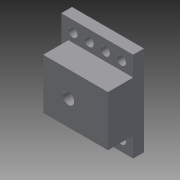
# Autodesk Inventor part: end limit holder
Saved by Autodesk Inventor 2013 SP2 (Build 170200200, 200)
## iProperties
Created: 2017-05-27
Part Number: end limit holder
Material: Generic
Document SubType Name: Modeling
Designer: hdv
Density: 1 g/cm^3
Author: hdv
Autodesk Inventor part; units mm, degrees
ref_plane "YZ Plane" through (0, 0, 0) normal (1, 0, 0) x (0, 1, 0)
ref_plane "XZ Plane" through (0, 0, 0) normal (0, 1, 0) x (-1, 0, 0)
ref_plane "XY Plane" through (0, 0, 0) normal (0, 0, 1) x (1, 0, 0)
sketch "Sketch1" plane through (0, 0, 0) normal (0, 0, 1) x (1, 0, 0)
  line L0 (0, 0) -> (20, 0)
  line L1 (20, 0) -> (20, 25)
  line L2 (20, 25) -> (0, 25)
  line L3 (0, 25) -> (0, 0)
  line L4 (5, 16.5) -> (17, 16.5)
  line L5 (17, 16.5) -> (17, 8.5)
  line L6 (17, 8.5) -> (5, 8.5)
  line L7 (5, 8.5) -> (5, 16.5)
  point P0 (17, 12.5)
  point P1 (20, 12.5)
  dimension "d0" = 20
  dimension "d2" = 25
  dimension "d3" = 8
  dimension "d4" = 12
  dimension "d5" = 3
  constraints: 16 end point, 4 parallel, 2 horizontal, 2 midpoint, 2 perpendicular, 1 horizontal alignment
  measures "d0" distance of L1.end L2.end
  measures "d2" distance of L0.end L1.end
  measures "d3" distance of L6.end L4.start
  measures "d4" distance of L5.end L6.end
  measures "d5" distance between parallel lines of L1 L5
extrude "Extrusion1" add sketch "Sketch1" along normal blind 3
sketch "Sketch2" plane through (0, 0, 3) normal (0, 0, 1) x (1, 0, 0)
  line L0 (17, 16.5) -> (17, 8.5) projected
  line L1 (17, 8.5) -> (5, 8.5) projected
  line L2 (5, 8.5) -> (5, 16.5) projected
  line L3 (5, 16.5) -> (17, 16.5) projected
  line L4 (20, 0) -> (20, 25) projected
  line L5 (20, 19.5) -> (20, 5.5)
  line L6 (20, 5.5) -> (2, 5.5)
  line L7 (2, 5.5) -> (2, 19.5)
  line L8 (2, 19.5) -> (20, 19.5)
  constraints: 8 end point, 1 collinear, 3 other
extrude "Extrusion2" add sketch "Sketch2" along normal blind 7
sketch "Sketch3" plane through (0, 0, 10) normal (0, 0, 1) x (1, 0, 0)
  line L0 (17, 8.5) -> (5, 8.5) projected
  line L1 (5, 8.5) -> (5, 16.5) projected
  line L2 (5, 16.5) -> (17, 16.5) projected
  line L3 (17, 16.5) -> (17, 8.5) projected
  point P0 (0, 0)
extrude "Extrusion3" add sketch "Sketch3" against normal blind 3
sketch "Sketch4" plane through (0, 0, 0) normal (0, 0, -1) x (-1, 0, 0)
  line L0 (0, 0) -> (-20, 0) projected
  line L1 (-20, 25) -> (0, 25) projected
  line L2 (-20, 0) -> (-20, 25) projected
  circle A0 centre (-16.75, 22) radius 1.25
  circle A1 centre (-12.25, 22) radius 1.25
  circle A2 centre (-7.75, 22) radius 1.25
  circle A3 centre (-3.25, 22) radius 1.25
  circle A4 centre (-16.75, 3) radius 1.25
  circle A5 centre (-12.25, 3) radius 1.25
  circle A6 centre (-7.75, 3) radius 1.25
  circle A7 centre (-3.25, 3) radius 1.25
  line L3 (-12.25, 22) -> (-7.75, 22)
  line L4 (-17, 8.5) -> (-17, 16.5) projected
  line L5 (-17, 16.5) -> (-5, 16.5) projected
  circle A8 centre (-9, 12.5) radius 1.6
  line L6 (-5, 16.5) -> (-5, 8.5) projected
  point P0 (-10, 22)
  point P1 (-10, 25)
  point P2 (-17, 12.5)
  point P3 (-11, 16.5)
  dimension "d12" = 2.5
  dimension "d13" = 2.5
  dimension "d14" = 2.5
  dimension "d15" = 2.5
  dimension "d16" = 2.5
  dimension "d17" = 2.5
  dimension "d18" = 2.5
  dimension "d19" = 2.5
  dimension "d20" = 4.5
  dimension "d21" = 4.5
  dimension "d22" = 4.5
  dimension "d23" = 3
  dimension "d24" = 3
  dimension "d27" = 3.2
  dimension "d28" = 4
  constraints: 9 centre point, 7 horizontal alignment, 5 vertical alignment, 4 midpoint, 2 end point, 1 perpendicular
  measures "d12" diameter of A0
  measures "d13" diameter of A1
  measures "d14" diameter of A2
  measures "d15" diameter of A3
  measures "d16" diameter of A4
  measures "d17" diameter of A5
  measures "d18" diameter of A6
  measures "d19" diameter of A7
  measures "d20" distance of L3.start A0.centre
  measures "d21" distance of L3.end L3.start
  measures "d22" distance of A3.centre L3.end
  measures "d23" distance from line of A0.centre L1
  measures "d24" distance from line of A4.centre L0
  measures "d27" diameter of A8
  measures "d28" distance from line of A8.centre L6
extrude "Extrusion4" cut sketch "Sketch4" against normal blind 10
equation "\"d21\" = d20"
equation "\"d22\" = d20"
equation "\"d24\" = d23"
body "Solid1"
